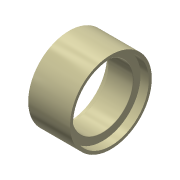
# Autodesk Inventor part: 3136 7009 52
Saved by Autodesk Inventor 2022 Beta2 (Build 260130000, 130) ContinuousBuild 0
## iProperties
Shininess: 31.0
Length Units: 11269
Angle Units: 11279
Time Units: 11290
Mass Units: 11283
Length Display Precision: 3
Angle Display Precision: 2
Compacted: True
Created: 2001-02-20
Part Number: 3136 7009 52
Document SubType Name: Modeling
Designer: Joe M
Material: Nylon 6/6
Description: Piston
Engineer: Joe M
Density: 1.13 g/cm^3
Appearance: Nylon 6
Density: 1.13
Volumn: 32.42050770303565
Area: 142.99987053837322
PropertySet Name: Model Information
Control State: 0
Master: False
Checked Out: False
Last Check In Date: 2001-02-28
Last Check In By: brpog
Title: Kolvtätning
Author: Joe M
Autodesk Inventor part; units mm, degrees
ref_plane "YZ Plane" through (0, 0, 0) normal (1, 0, 0) x (0, 1, 0)
ref_plane "XZ Plane" through (0, 0, 0) normal (0, 1, 0) x (-1, 0, 0)
ref_plane "XY Plane" through (0, 0, 0) normal (0, 0, 1) x (1, 0, 0)
sketch "Sketch1" plane through (0, 0, 0) normal (0, 0, 1) x (1, 0, 0)
  line L0 (0, 23.5) -> (9.3, 23.5)
  line L1 (9.7, 23.9) -> (9.7, 29.2)
  line L2 (9.7, 29.2) -> (16.1, 29.2)
  line L3 (16.1, 29.2) -> (16.1, 31.5)
  line L4 (16.1, 31.5) -> (0, 31.5)
  line L5 (0, 23.5) -> (0, 39.7331)
  arc A0 (9.3, 23.5) -> (9.7, 23.9) centre (9.3, 23.9) ccw
  line L6 (0, 0) -> (48.7382, 0)
  line L7 (0, 23.5) -> (-9.3, 23.5)
  line L8 (-9.7, 23.9) -> (-9.7, 29.2)
  line L9 (-9.7, 29.2) -> (-16.1, 29.2)
  line L10 (-16.1, 29.2) -> (-16.1, 31.5)
  line L11 (-16.1, 31.5) -> (0, 31.5)
  arc A1 (-9.7, 23.9) -> (-9.3, 23.5) centre (-9.3, 23.9) ccw
  dimension "d0" = 0.4
  dimension "d1" = 47
  dimension "d2" = 63
  dimension "d3" = 58.4
  dimension "d4" = 16.1
  dimension "d5" = 9.7
  constraints: 24 end point, 6 symmetric about line, 4 perpendicular, 4 point on circle, 3 parallel, 2 centre point, 2 tangent, 1 coincident, 1 horizontal, 1 point on line, 1 vertical alignment, 6 other
  measures "d0" radius of A0
  measures "d1" diameter of L0 L6
  measures "d2" diameter of L4 L6
  measures "d3" diameter of L2 L6
  measures "d4" distance of L3.end L4.end
  measures "d5" distance from line of L0.start L1
revolve "Revolution1" add sketch "Sketch1" angle 360 about axis through (0, 0, 0) along (1, 0, 0)
body "Solid1"
